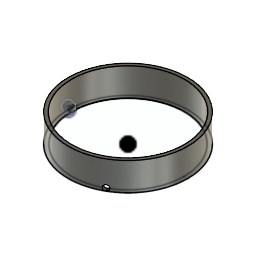
outer_mount (Autodesk Fusion 360 design; units mm, degrees)
part number: 2025-12-16-22-53-18-255
Autodesk Fusion 360 part; units mm, degrees
sketch "Sketch1" plane through (0, 0, 0) normal (0, 0, 1) x (1, 0, 0)
  circle A0 centre (0, 0) radius 30
  circle A1 centre (0, 0) radius 32
  dimension "d1" = 60
  dimension "d2" = 64
  constraint coincident A0.centre A1.centre
  constraint concentric A0 A1
  measures "d1" diameter of A0
  measures "d2" diameter of A1
extrude "Extrude1" add sketch "Sketch1" along normal blind 15
ref_plane "WorkPlane1" through (-32, 0, 6.0325) normal (-1, 0, 0) x (0, 1, 0)
sketch "Sketch2" plane through (-32, 0, 0) normal (-1, 0, 0) x (0, -1, 0)
  line L0 (0, 0) -> (0, 1.5)
  circle A0 centre (0, 1.5) radius 1.5
  constraint coincident L0.start origin
  constraint vertical L0
  constraint coincident L0.end A0.centre
  constraint coincident L0.start A0
extrude "Extrude2" cut sketch "Sketch2" against normal blind 4
move_face "OffsetFaces1" offset -0.25 1 faces at (-25.5987, -15.6431, 5)
pattern_circular "C-Pattern1" count 3 over 360 about axis through (0, 0, 1.75) along (0, 0, 1) of "Extrude2"
